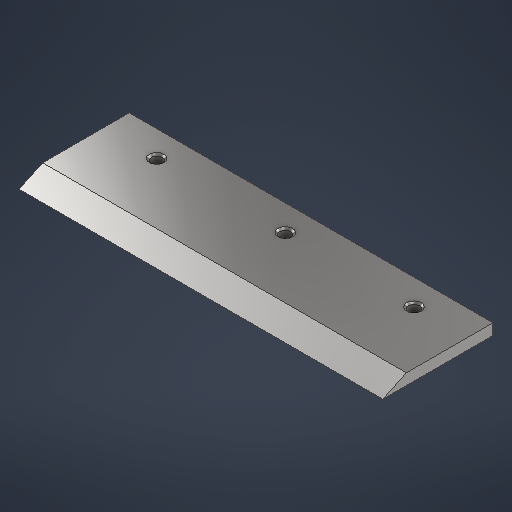
# Autodesk Inventor part: Knife
Saved by Autodesk Inventor 2027 (Build 310192000, 192)
## iProperties
Created: 2026-04-01
Part Number: Knife
Material: Ocel, uhlík
Document SubType Name: Modeling
Designer: Vadim Sobčuk
Density: 7.85 g/cm^3
Appearance: Pololeštěná
Checked By: Vadim Sobčuk
Engr Approved By: Vadim Sobčuk
Mfg Approved By: Vadim Sobčuk
Engineer: Vadim Sobčuk
Authority: Vadim Sobčuk
Author: Vadaim Sobčuk
Title: Knife
Autodesk Inventor part; units mm, degrees
ref_plane "YZ Plane" through (0, 0, 0) normal (1, 0, 0) x (0, 1, 0)
ref_plane "XZ Plane" through (0, 0, 0) normal (0, 1, 0) x (-1, 0, 0)
ref_plane "XY Plane" through (0, 0, 0) normal (0, 0, 1) x (1, 0, 0)
sketch "Náčrt1" plane through (0, 0, 0) normal (1, 0, 0) x (0, 1, 0)
  line L0 (1.5, 15) -> (-1.5, 15)
  line L1 (-1.5, 15) -> (-1.5, -15)
  line L2 (-1.5, -15) -> (1.5, -15)
  line L3 (1.5, -15) -> (1.5, 15)
  line L4 (1.5, 15) -> (-1.5, -15) construction
  line L5 (-1.5, 15) -> (1.5, -15) construction
  line L6 (-1.5, 15) -> (1.5, 8.5665)
  point P0 (0, 0)
  dimension "d0" = 3
  dimension "d1" = 30
  dimension "d2" = 25
  constraints: 14 end point, 2 midpoint, 2 parallel, 1 horizontal, 1 perpendicular, 1 point on line
  measures "d0" distance between parallel lines of L1 L3
  measures "d1" distance between parallel lines of L0 L2
  measures "d2" angle of L1 L6
extrude "Vysunutí1" add sketch "Náčrt1" along normal mid plane 99 contours L6 L3 L2 L1
sketch "Náčrt2" plane through (-49.5, -1.5, -15) normal (0, -1, 0) x (1, 0, 0)
  circle A0 centre (84.5, 7) radius 1.5
  circle A1 centre (49.5, 7) radius 1.5
  circle A2 centre (14.5, 7) radius 1.5
  line L0 (0, 0) -> (99, 0) projected
  line L1 (99, 30) -> (99, 0) projected
  line L2 (0, 30) -> (99, 30) projected
  line L3 (0, 0) -> (0, 30) projected
  line L4 (99, 7) -> (0, 7) construction
  line L5 (49.5, 0) -> (49.5, 30) construction
  point P0 (49.5, 15)
  dimension "d5" = 7
  dimension "d6" = 3
  dimension "d7" = 35
  dimension "d8" = 3
  constraints: 4 end point, 4 point on line, 3 centre point, 3 midpoint, 1 coincident, 1 perpendicular, 1 other
  measures "d5" distance between parallel lines of L0 L4
  measures "d6" diameter of A1
  measures "d7" distance of A1.centre A2.centre
  measures "d8" diameter of A2
extrude "Vysunutí2" cut sketch "Náčrt2" against normal through all contours A0 | A1 | A2
thread "Závit1" size "M3x0.5" class "6H" standard "ANSI Metric M Profile" full length
thread "Závit2" size "M3x0.5" class "6H" standard "ANSI Metric M Profile" full length
thread "Závit3" size "M3x0.5" class "6H" standard "ANSI Metric M Profile" full length
chamfer "Zkosení1" distance 0.5 angle 45 3 edges at (-36.5, 1.5, -8) (-1.5, 1.5, -8) (33.5, 1.5, -8)
sketch "Náčrt3" plane through (-49.5, -1.5, -15) normal (0, -1, 0) x (1, 0, 0)
  circle A0 centre (14.5, 7) radius 1.5 projected
  circle A1 centre (49.5, 7) radius 1.5 projected
  circle A2 centre (84.5, 7) radius 1.5 projected
  line L0 (0, 0) -> (99, 0) projected
  line L1 (99, 30) -> (99, 0) projected
  line L2 (0, 30) -> (99, 30) projected
  line L3 (0, 0) -> (0, 30) projected
  line L4 (98.5, 0.5) -> (53.2335, 0.5) construction
  line L5 (53.2335, 0.5) -> (53.2335, 9.4631) construction
  line L6 (53.2335, 9.4631) -> (98.5, 9.4631) construction
  line L7 (98.5, 9.4631) -> (98.5, 0.5) construction
  point P0 (49.5, 15)
  dimension "d0" = 3
  dimension "d1" = 30
  dimension "d2" = 25
  dimension "d22" = 0.5
  dimension "d23" = 0.5
  constraints: 2 other
  measures "d22" distance between parallel lines of L0 L4
  measures "d23" distance between parallel lines of L1 L7
